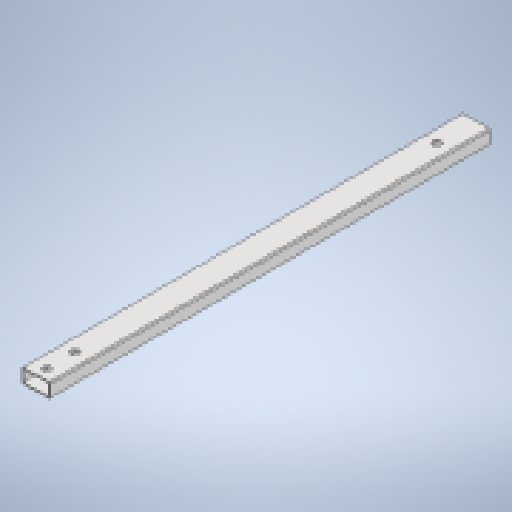
# Autodesk Inventor part: Short tube 3
Saved by Autodesk Inventor 2026.2 (Build 302298000, 298)
## iProperties
Created: 2026-05-21
Part Number: Short tube 3
Material: Generic
Document SubType Name: Modeling
Designer: admin
Density: 1 g/cm^3
Appearance: Default
Author: admin
Autodesk Inventor part; units mm, degrees
ref_plane "YZ Plane" through (0, 0, 0) normal (1, 0, 0) x (0, 1, 0)
ref_plane "XZ Plane" through (0, 0, 0) normal (0, 1, 0) x (-1, 0, 0)
ref_plane "XY Plane" through (0, 0, 0) normal (0, 0, 1) x (1, 0, 0)
sketch "Sketch1" plane through (0, 0, 0) normal (0, 0, 1) x (1, 0, 0)
  line L0 (-20, 10) -> (20, 10)
  line L1 (20, 10) -> (20, -10)
  line L2 (20, -10) -> (-20, -10)
  line L3 (-20, -10) -> (-20, 10)
  line L4 (-20, 10) -> (20, -10) construction
  line L5 (20, 10) -> (-20, -10) construction
  line L6 (18, 8) -> (-18, 8)
  line L7 (-18, 8) -> (-18, -8)
  line L8 (-18, -8) -> (18, -8)
  line L9 (18, -8) -> (18, 8)
  point P0 (0, 0)
  dimension "d0" = 40
  dimension "d1" = 20
  dimension "d2" = 2
  constraints: 20 end point, 4 parallel, 2 midpoint, 2 perpendicular, 1 horizontal, 3 other
  measures "d0" distance of L1.end L2.end
  measures "d1" distance of L0.end L1.end
  measures "d2" distance between parallel lines of L0 L6
extrude "Extrusion1" add sketch "Sketch1" along normal mid plane 620
fillet "Fillet1" radius 2 4 edges at (-20, 10, 0) (-20, -10, 0) (20, -10, 0) (20, 10, 0)
sketch "Sketch4" plane through (0, 0, 0) normal (0, 1, 0) x (-1, 0, 0)
  circle A0 centre (0, -255) radius 5.5
  circle A1 centre (0, 255) radius 5.5
  line L0 (46.2729, 0) -> (-46.2729, 0) construction
  line L1 (-18, 310) -> (18, 310) projected
  circle A2 centre (0, 295) radius 5.5
  point P0 (0, 0)
  point P1 (0, 0)
  point P2 (0, 310)
  dimension "d20" = 11
  dimension "d21" = 55
  dimension "d24" = 40
  constraints: 3 centre point, 2 end point, 2 equal radius, 2 midpoint, 2 vertical alignment, 1 coincident, 1 horizontal, 1 other
  measures "d20" diameter of A1
  measures "d21" distance from line of L1 A1.centre
  measures "d24" distance of A2.centre A1.centre
extrude "Extrusion4" cut sketch "Sketch4" along normal through all
body "Solid1"
